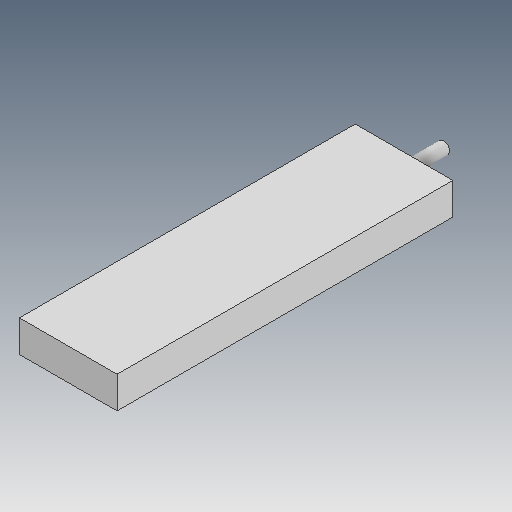
# Autodesk Inventor part: anker_4-port_usb3.0_splitter
Saved by Autodesk Inventor 2025.4 (Build 294407020, 407B)
## iProperties
Created: 2026-09-16
Part Number: anker_4-port_usb3.0_splitter
Material: Generic
Document SubType Name: Modeling
Designer: Aiden
Density: 1 g/cm^3
Appearance: Default
Author: Aiden
Autodesk Inventor part; units mm, degrees
ref_plane "YZ Plane" through (0, 0, 0) normal (1, 0, 0) x (0, 1, 0)
ref_plane "XZ Plane" through (0, 0, 0) normal (0, 1, 0) x (-1, 0, 0)
ref_plane "XY Plane" through (0, 0, 0) normal (0, 0, 1) x (1, 0, 0)
sketch "Sketch1" plane through (0, 0, 0) normal (0, 1, 0) x (-1, 0, 0)
  line L0 (15.621, 53.721) -> (-15.621, 53.721)
  line L1 (-15.621, 53.721) -> (-15.621, -53.721)
  line L2 (-15.621, -53.721) -> (15.621, -53.721)
  line L3 (15.621, -53.721) -> (15.621, 53.721)
  line L4 (15.621, 53.721) -> (-15.621, -53.721) construction
  line L5 (-15.621, 53.721) -> (15.621, -53.721) construction
  point P0 (0, 0)
  dimension "d0" = 107.442
  dimension "d1" = 31.242
  constraints: 12 end point, 2 midpoint, 2 parallel, 1 horizontal, 1 perpendicular
  measures "d0" distance of L0.end L1.end
  measures "d1" distance of L1.end L2.end
extrude "Extrusion1" add sketch "Sketch1" along normal blind 10.16
sketch "Sketch2" plane through (-15.621, 0, -53.721) normal (-1, 0, 0) x (0, 0, 1)
  line L0 (0, 0) -> (0, 10.16) projected
  line L1 (0, 5.08) -> (107.442, 5.08) construction
  line L2 (107.442, 0) -> (107.442, 10.16) projected
  line L3 (107.442, 10.16) -> (0, 10.16) projected
  line L4 (53.721, 10.16) -> (53.721, 0) construction
  line L5 (107.442, 0) -> (0, 0) projected
  line L6 (35.2574, 2.1925) -> (48.2344, 2.1925)
  line L7 (48.2344, 2.1925) -> (48.2344, 7.9675)
  line L8 (48.2344, 7.9675) -> (35.2574, 7.9675)
  line L9 (35.2574, 7.9675) -> (35.2574, 2.1925)
  line L10 (35.2574, 2.1925) -> (48.2344, 7.9675) construction
  line L11 (48.2344, 2.1925) -> (35.2574, 7.9675) construction
  line L12 (0, 10.16) -> (53.721, 10.16)
  line L13 (26.8605, 10.16) -> (26.8605, 0) construction
  line L14 (18.4636, 2.1925) -> (5.4866, 2.1925)
  line L15 (5.4866, 2.1925) -> (5.4866, 7.9675)
  line L16 (5.4866, 7.9675) -> (18.4636, 7.9675)
  line L17 (18.4636, 7.9675) -> (18.4636, 2.1925)
  line L18 (18.4636, 2.1925) -> (5.4866, 7.9675) construction
  line L19 (5.4866, 2.1925) -> (18.4636, 7.9675) construction
  line L20 (107.442, 5.08) -> (0, 5.08) construction
  line L21 (72.1846, 2.1925) -> (59.2076, 2.1925)
  line L22 (59.2076, 2.1925) -> (59.2076, 7.9675)
  line L23 (59.2076, 7.9675) -> (72.1846, 7.9675)
  line L24 (72.1846, 7.9675) -> (72.1846, 2.1925)
  line L25 (72.1846, 2.1925) -> (59.2076, 7.9675) construction
  line L26 (59.2076, 2.1925) -> (72.1846, 7.9675) construction
  line L27 (80.5815, 10.16) -> (80.5815, 0) construction
  line L28 (88.9784, 2.1925) -> (101.9554, 2.1925)
  line L29 (101.9554, 2.1925) -> (101.9554, 7.9675)
  line L30 (101.9554, 7.9675) -> (88.9784, 7.9675)
  line L31 (88.9784, 7.9675) -> (88.9784, 2.1925)
  line L32 (88.9784, 2.1925) -> (101.9554, 7.9675) construction
  line L33 (101.9554, 2.1925) -> (88.9784, 7.9675) construction
  point P0 (41.7459, 5.08)
  point P1 (11.9751, 5.08)
  point P2 (65.6961, 5.08)
  point P3 (95.4669, 5.08)
  constraints: 60 end point, 19 symmetric about line, 6 midpoint, 4 perpendicular, 3 point on line, 2 parallel, 1 horizontal
extrude "Extrusion2" cut sketch "Sketch2" against normal blind 10.16 contours L9 L8 L7 L6 | L14 L15 L16 L17 | L21 L22 L23 L24 | L31 L30 L29 L28
sketch "Sketch3" plane through (15.621, 0, -53.721) normal (0, 0, -1) x (-1, 0, 0)
  line L0 (0, 10.16) -> (31.242, 10.16) projected
  line L1 (15.621, 10.16) -> (15.621, 0) construction
  circle A0 centre (15.621, 5.08) radius 1.905
  dimension "d6" = 3.81
  constraints: 2 end point, 2 midpoint, 1 centre point, 1 vertical
  measures "d6" diameter of A0
extrude "Extrusion3" add sketch "Sketch3" along normal blind 12.7
body "Solid1"
